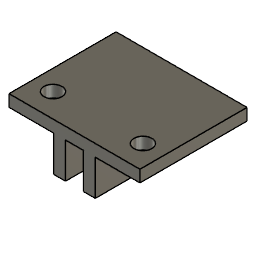
soporte sensor_ (Autodesk Fusion 360 design; units mm, degrees)
Autodesk Fusion 360 part; units mm, degrees
sketch "Boceto1" plane through (0, 0, 0) normal (0, 0, 1) x (1, 0, 0)
  line L0 (0, 0) -> (22, 0)
  line L1 (22, 0) -> (22, 18)
  line L2 (22, 18) -> (0, 18)
  line L3 (0, 18) -> (0, 0)
  dimension "d3" = 22
  dimension "d4" = 18
  constraint horizontal L0
  constraint vertical L1
  constraint horizontal L2
  constraint vertical L3
  constraint coincident L0.start L3.end
  measures "d3" distance of L0.start L0.end
  measures "d4" distance of L0.start L2.end
extrude "Extruir1" add sketch "Boceto1" along normal blind 2
sketch "Boceto2" plane through (0, 0, 0) normal (0, 0, -1) x (1, 0, 0)
  line L0 (0, 0) -> (0, -18)
  line L1 (0, -18) -> (22, -18)
  line L2 (22, -18) -> (22, 0)
  line L3 (22, 0) -> (0, 0)
  line L4 (7.5, 0) -> (9.5, 0)
  line L5 (9.5, 0) -> (9.5, -18)
  line L6 (9.5, -18) -> (7.5, -18)
  line L7 (7.5, -18) -> (7.5, 0)
  line L8 (14.5, 0) -> (12.5, 0)
  line L9 (12.5, 0) -> (12.5, -18)
  line L10 (12.5, -18) -> (14.5, -18)
  line L11 (14.5, -18) -> (14.5, 0)
  dimension "d7" = 2
  dimension "d8" = 2
  constraint coincident L3 L4.start
  constraint horizontal L4
  constraint vertical L5
  constraint horizontal L6
  constraint vertical L7
  constraint horizontal L8
  constraint vertical L9
  constraint horizontal L10
  constraint vertical L11
  measures "d7" distance of L4.start L4.end
  measures "d8" distance of L8.start L8.end
extrude "Extruir2" add sketch "Boceto2" along normal blind 6 contours L1 L3 L4 L5 L6 L7 | L1 L3 L8 L9 L10 L11
sketch "Boceto3" plane through (14.5, 0, 0) normal (1, 0, 0) x (0, 1, 0)
  line L0 (18, 0) -> (0, 0)
  line L1 (0, 0) -> (0, -6)
  line L2 (0, -6) -> (18, -6)
  line L3 (18, -6) -> (18, 0)
  circle A0 centre (9, -3) radius 1.5
  dimension "d11" = 3
  measures "d11" diameter of A0
extrude "Extruir3" cut sketch "Boceto3" against normal blind 7 contours A0
sketch "Boceto4" plane through (0, 0, 2) normal (0, 0, 1) x (-1, 0, 0)
  line L0 (0, -18) -> (0, 0)
  line L1 (0, 0) -> (-22, 0)
  line L2 (-22, 0) -> (-22, -18)
  line L3 (-22, -18) -> (0, -18)
  circle A0 centre (-3.4, -4) radius 1.5
  circle A1 centre (-18.5, -4) radius 1.5
  dimension "d14" = 3
  dimension "d15" = 3
  measures "d14" diameter of A0
  measures "d15" diameter of A1
extrude "Extruir4" cut sketch "Boceto4" against normal blind 2 contours A0 | A1
